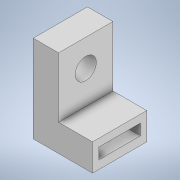
# Autodesk Inventor part: axelAdjustment 1-13
Saved by Autodesk Inventor 2020 (Build 240168000, 168)
## iProperties
Created: 2020-01-14
Part Number: axelAdjustment 1-13
Material: Generic
Document SubType Name: Modeling
Designer: akend
Density: 1 g/cm^3
Appearance: Default
Author: akend
## iProperties of the stored document _3DPrint.ipt
Created: 2020-01-14
Part Number: _3DPrint
Material: Generic
Document SubType Name: Modeling
Designer: akend
Density: 1 g/cm^3
Appearance: Default
Author: akend
Autodesk Inventor part; units mm, degrees
ref_plane "YZ Plane" through (0, 0, 0) normal (1, 0, 0) x (0, 1, 0)
ref_plane "XZ Plane" through (0, 0, 0) normal (0, 1, 0) x (-1, 0, 0)
ref_plane "XY Plane" through (0, 0, 0) normal (0, 0, 1) x (1, 0, 0)
sketch "Sketch1" plane through (0, 0, 0) normal (1, 0, 0) x (0, 1, 0)
  line L0 (0, 0) -> (25.75, 0)
  line L1 (25.75, 0) -> (25.75, -16)
  line L2 (25.75, -16) -> (0, -16)
  line L3 (0, -16) -> (0, 0)
  line L4 (0, 0) -> (2.5, 0) construction
  line L5 (2.5, 0) -> (2.5, -16) construction
  line L6 (2.5, -16) -> (0, -16) construction
  line L7 (0, -16) -> (0, 0) construction
  line L8 (0, 0) -> (1.875, 0) construction
  line L9 (0, -2.8568) -> (0, 0) construction
  line L10 (0, 0) -> (25.75, 0) construction
  line L11 (25.75, 0) -> (25.75, -1.875) construction
  line L12 (25.75, -1.875) -> (0, -1.875) construction
  line L13 (0, -1.875) -> (0, 0) construction
  line L14 (25.75, -16) -> (0, -16) construction
  line L15 (0, -16) -> (0, -14.125) construction
  line L16 (0, -14.125) -> (25.75, -14.125) construction
  line L17 (25.75, -14.125) -> (25.75, -16) construction
  line L18 (2.5, -1.875) -> (5.75, -1.875)
  line L19 (5.75, -1.875) -> (5.75, -14.125)
  line L20 (5.75, -14.125) -> (2.5, -14.125)
  line L21 (2.5, -14.125) -> (2.5, -1.875)
  circle A0 centre (17.75, -8) radius 3.125
  dimension "d0" = 25.75
  dimension "d1" = 16
  dimension "d2" = 2.5
  dimension "d4" = 1.875
  dimension "d5" = 1.875
  dimension "d6" = 3.25
  dimension "d7" = 6.25
  constraints: 44 end point, 10 parallel, 6 horizontal, 6 point on line, 5 perpendicular, 1 centre point
  measures "d0" distance of L1.end L2.end
  measures "d1" distance of L0.end L1.end
  measures "d2" distance of L5.end L6.end
  measures "d4" distance of L10.end L11.end
  measures "d5" distance of L14.end L15.end
  measures "d6" distance of L19.end L20.end
  measures "d7" diameter of A0
extrude "Extrusion1" add sketch "Sketch1" along normal blind 7.5
sketch "Sketch2" plane through (7.5, 0, 0) normal (1, 0, 0) x (0, 0, -1)
  line L0 (0, 0) -> (16, 0) projected
  line L1 (16, 0) -> (16, 25.75) projected
  line L2 (0, 0) -> (16, 0)
  line L3 (16, 0) -> (16, 8)
  line L4 (16, 8) -> (0, 8)
  line L5 (0, 8) -> (0, 0)
  line L6 (1.875, 2.5) -> (1.875, 5.75) projected
  line L7 (14.125, 5.75) -> (14.125, 2.5) projected
  line L8 (1.875, 5.75) -> (14.125, 5.75)
  line L9 (14.125, 5.75) -> (14.125, 2.5)
  line L10 (14.125, 2.5) -> (1.875, 2.5)
  line L11 (1.875, 2.5) -> (1.875, 5.75)
  dimension "d10" = 8
  constraints: 16 end point, 4 parallel, 2 horizontal, 2 perpendicular, 1 point on line
  measures "d10" distance of L3.end L2.end
extrude "Extrusion2" add sketch "Sketch2" along normal blind 10
body "Solid1"
